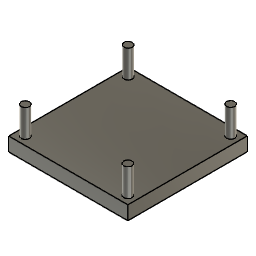
reggiL298N (Autodesk Fusion 360 design; units mm, degrees)
part number: 2025-07-05-13-01-11-481
Autodesk Fusion 360 part; units mm, degrees
note: some values were not read from the file. Set by a fixed rule: which sketch regions a step uses.
sketch "Schizzo1" plane through (0, 0, 0) normal (0, 0, 1) x (1, 0, 0)
  line L0 (0, 0) -> (43.2, 0)
  line L1 (43.2, 0) -> (43.2, 43.3)
  line L2 (43.2, 43.3) -> (0, 43.3)
  line L3 (0, 43.3) -> (0, 0)
  line L4 (0, 0) -> (0, 1.5)
  line L5 (0, 43.3) -> (0, 41.8)
  line L6 (0, 43.3) -> (1.5, 43.3)
  line L7 (43.2, 43.3) -> (41.7, 43.3)
  line L8 (0, 1.5) -> (0, 3)
  line L9 (0, 43.3) -> (0, 40.3)
  line L10 (1.5, 43.3) -> (3, 43.3)
  line L11 (43.2, 43.3) -> (40.2, 43.3)
  line L12 (3, 43.3) -> (3, 0)
  line L13 (0, 3) -> (43.2, 3)
  line L14 (0, 40.3) -> (43.2, 40.3)
  line L15 (40.2, 43.3) -> (40.2, 0)
  circle A0 centre (3, 40.3) radius 1.5
  circle A1 centre (40.2, 40.3) radius 1.5
  circle A2 centre (3, 3) radius 1.5
  circle A3 centre (40.2, 3) radius 1.5
  dimension "d1" = 43.2
  dimension "d2" = 43.3
  dimension "d3" = 1.5
  dimension "d4" = 1.5
  dimension "d5" = 1.5
  dimension "d6" = 1.5
  dimension "d7" = 1.5
  dimension "d8" = 3
  dimension "d9" = 1.5
  dimension "d10" = 3
  dimension "d11" = 3
  dimension "d12" = 3
  dimension "d13" = 3
  dimension "d14" = 3
  constraint horizontal L0
  constraint vertical L1
  constraint horizontal L2
  constraint vertical L3
  constraint coincident L0.start L3.end
  constraint perpendicular L0 L4
  constraint perpendicular L2 L5
  constraint perpendicular L3 L6
  constraint perpendicular L1 L7
  constraint perpendicular L0 L8
  constraint perpendicular L6 L9
  constraint perpendicular L3 L10
  constraint perpendicular L1 L11
  constraint coincident L0 L12.end
  constraint perpendicular L0 L12
  constraint coincident L1 L13.end
  constraint perpendicular L1 L13
  constraint coincident L1 L14.end
  constraint perpendicular L1 L14
  constraint coincident L0 L15.end
  constraint perpendicular L0 L15
  constraint coincident L12 A0.centre
  constraint coincident L14 A0.centre
  constraint coincident L14 A1.centre
  constraint coincident L15 A1.centre
  constraint coincident L13 A2.centre
  constraint coincident L12 A2.centre
  constraint coincident L15 A3.centre
  constraint coincident L13 A3.centre
  measures "d1" distance of L0.start L0.end
  measures "d2" distance of L0.start L2.end
  measures "d3" distance of L0.start L4.end
  measures "d4" distance of L2.end L5.end
  measures "d5" distance of L2.end L6.end
  measures "d6" distance of L1.end L7.end
  measures "d7" distance of L4.end L8.end
  measures "d8" distance of L2.end L9.end
  measures "d9" distance of L6.end L10.end
  measures "d10" distance of L1.end L11.end
  measures "d11" diameter of A0
  measures "d12" diameter of A1
  measures "d13" diameter of A2
  measures "d14" diameter of A3
extrude "Estrusione1" add sketch "Schizzo1" along normal blind 15 contours L12 L13 A2 | L12 L13 A2 | L13 L15 A3 | L13 L15 A3 | L12 L13 A2 | L12 L13 A2 | L13 L15 A3 | L13 L15 A3 | L12 L14 A0 | L12 L14 A0 | L12 L14 A0 | L12 L14 A0 | L14 L15 A1 | L14 L15 A1 | L14 L15 A1 | L14 L15 A1 makes body 1 at (1.6178, 40.8827, 10) makes body 2 at (41.5173, 41.0174, 5) makes body 3 at (4.4925, 2.8506, 5) makes body 4 at (41.0756, 1.7821, 10)
sketch "Schizzo2" plane through (0, 0, 0) normal (0, 0, 1) x (1, 0, 0)
  line L0 (0, 0) -> (43.2, 0)
  line L1 (43.2, 0) -> (43.2, 43.3)
  line L2 (43.2, 43.3) -> (0, 43.3)
  line L3 (0, 43.3) -> (0, 0)
  dimension "d17" = 43.2
  dimension "d18" = 43.3
  constraint horizontal L0
  constraint vertical L1
  constraint horizontal L2
  constraint vertical L3
  constraint coincident L0.start L3.end
  measures "d17" distance of L0.start L0.end
  measures "d18" distance of L0.start L2.end
extrude "Estrusione2" add sketch "Schizzo2" along normal blind 5 bodies 1 2 3 4
